Autodesk Fusion 360 part; units mm, degrees
(part 5 of 7)
sketch "Full-depth inlet-to-outlet bypass barrier sketch" plane through (0, 0, 4.9) normal (0, 0, 1) x (1, 0, 0) in component "Chamber / A3 top manifold with serial return"
  line L0 (4.9, 158) -> (27.25, 158)
  line L1 (27.25, 158) -> (27.25, 162.6)
  line L2 (27.25, 162.6) -> (4.9, 162.6)
  line L3 (4.9, 162.6) -> (4.9, 158)
  dimension "d1577" = 4.9
  dimension "d1578" = 158
  dimension "d1579" = 22.35
  dimension "d1580" = 4.6
  constraint horizontal L0
  constraint vertical L1
  constraint horizontal L2
  constraint vertical L3
  measures "d1577" horizontal distance of origin L0.start
  measures "d1578" vertical distance of origin L0.start
  measures "d1579" horizontal distance of L0.start L0.end
  measures "d1580" vertical distance of L0.end L1.end
extrude "Full-depth inlet-to-outlet bypass barrier" add sketch "Full-depth inlet-to-outlet bypass barrier sketch" along normal blind 31.1 contours L0 L1 L2 L3 picked at (12.35, 161.066667) bodies 74 in component "Chamber / A3 top manifold with serial return"
ref_plane "WorkPlane9" through (0, 0, 4.9) normal (0, 0, 1) x (1, 0, 0) in component "Chamber / A3 top manifold with serial return"
sketch "Exhaust junction upper 2 mm wall extension sketch" plane through (0, 0, 4.9) normal (0, 0, 1) x (1, 0, 0) in component "Chamber / A3 top manifold with serial return"
  line L0 (4.9, 162.5) -> (12.1, 162.5)
  line L1 (12.1, 162.5) -> (12.1, 167)
  line L2 (12.1, 167) -> (4.9, 167)
  line L3 (4.9, 167) -> (4.9, 162.5)
  dimension "d1585" = 4.9
  dimension "d1586" = 162.5
  dimension "d1587" = 7.2
  dimension "d1588" = 4.5
  constraint horizontal L0
  constraint vertical L1
  constraint horizontal L2
  constraint vertical L3
  measures "d1585" horizontal distance of origin L0.start
  measures "d1586" vertical distance of origin L0.start
  measures "d1587" horizontal distance of L0.start L0.end
  measures "d1588" vertical distance of L0.end L1.end
extrude "Exhaust junction upper 2 mm wall extension" add sketch "Exhaust junction upper 2 mm wall extension sketch" along normal blind 31.1 contours L0 L1 L2 L3 picked at (9.7, 164) bodies 74 in component "Chamber / A3 top manifold with serial return"
ref_plane "WorkPlane10" through (0, 0, 29) normal (0, 0, 1) x (1, 0, 0) in component "Chamber / A3 top manifold with serial return"
sketch "Rear return isolation above sensing-face sweep sketch" plane through (0, 0, 29) normal (0, 0, 1) x (1, 0, 0) in component "Chamber / A3 top manifold with serial return"
  line L0 (4.9, 149) -> (27.25, 149)
  line L1 (27.25, 149) -> (27.25, 158.1)
  line L2 (27.25, 158.1) -> (4.9, 158.1)
  line L3 (4.9, 158.1) -> (4.9, 149)
  dimension "d1593" = 4.9
  dimension "d1594" = 149
  dimension "d1595" = 22.35
  dimension "d1596" = 9.1
  constraint horizontal L0
  constraint vertical L1
  constraint horizontal L2
  constraint vertical L3
  measures "d1593" horizontal distance of origin L0.start
  measures "d1594" vertical distance of origin L0.start
  measures "d1595" horizontal distance of L0.start L0.end
  measures "d1596" vertical distance of L0.end L1.end
extrude "Rear return isolation above sensing-face sweep" add sketch "Rear return isolation above sensing-face sweep sketch" along normal blind 7 contours L0 L1 L2 L3 picked at (12.35, 152.033333) bodies 74 in component "Chamber / A3 top manifold with serial return"
ref_plane "WorkPlane11" through (0, 0, 28) normal (0, 0, 1) x (1, 0, 0) in component "Chamber / A3 top manifold with serial return"
sketch "Humidity compartment rear bypass baffle sketch" plane through (0, 0, 28) normal (0, 0, 1) x (1, 0, 0) in component "Chamber / A3 top manifold with serial return"
  line L0 (48, 162.4) -> (50, 162.4)
  line L1 (50, 162.4) -> (50, 175.1)
  line L2 (50, 175.1) -> (48, 175.1)
  line L3 (48, 175.1) -> (48, 162.4)
  dimension "d1601" = 48
  dimension "d1602" = 162.4
  dimension "d1603" = 2
  dimension "d1604" = 12.7
  constraint horizontal L0
  constraint vertical L1
  constraint horizontal L2
  constraint vertical L3
  measures "d1601" horizontal distance of origin L0.start
  measures "d1602" vertical distance of origin L0.start
  measures "d1603" horizontal distance of L0.start L0.end
  measures "d1604" vertical distance of L0.end L1.end
extrude "Humidity compartment rear bypass baffle" add sketch "Humidity compartment rear bypass baffle sketch" along normal blind 8 contours L0 L1 L2 L3 picked at (48.666667, 166.633333) bodies 74 in component "Chamber / A3 top manifold with serial return"
ref_plane "WorkPlane12" through (70.65, 0, 0) normal (1, 0, 0) x (0, 1, 0) in component "Chamber / A3 top manifold with serial return"
sketch "Inlet bore sketch" plane through (70.65, 0, 0) normal (1, 0, 0) x (0, 0, -1) in component "Chamber / A3 top manifold with serial return"
  circle A0 centre (-22, 162.5) radius 2.5
  dimension "d1610" = 162.5
  dimension "d1611" = 2.5
  measures "d1610" vertical distance of origin A0.centre
  measures "d1611" radius of A0
extrude "Inlet bore" cut sketch "Inlet bore sketch" along normal blind 11.45 contours A0 picked at (-21.937725, 164.26987) bodies 74 in component "Chamber / A3 top manifold with serial return"
ref_plane "WorkPlane13" through (0, 162.4, 0) normal (0, 1, 0) x (0, 0, 1) in component "Chamber / A3 top manifold with serial return"
sketch "Inlet rise bore sketch" plane through (0, 162.4, 0) normal (0, 1, 0) x (1, 0, 0) in component "Chamber / A3 top manifold with serial return"
  circle A0 centre (70.75, -22) radius 2.5
  dimension "d1616" = 70.75
  dimension "d1618" = 2.5
  measures "d1616" horizontal distance of origin A0.centre
  measures "d1618" radius of A0
extrude "Inlet rise bore" cut sketch "Inlet rise bore sketch" along normal blind 2.7 contours A0 picked at (70.581043, -23.369363) bodies 74 in component "Chamber / A3 top manifold with serial return"
ref_plane "WorkPlane14" through (67.9, 0, 0) normal (1, 0, 0) x (0, 1, 0) in component "Chamber / A3 top manifold with serial return"
sketch "Upper inlet turn bore sketch" plane through (67.9, 0, 0) normal (1, 0, 0) x (0, 0, -1) in component "Chamber / A3 top manifold with serial return"
  circle A0 centre (-22, 165) radius 2.5
  dimension "d1624" = 165
  dimension "d1625" = 2.5
  measures "d1624" vertical distance of origin A0.centre
  measures "d1625" radius of A0
extrude "Upper inlet turn bore" cut sketch "Upper inlet turn bore sketch" along normal blind 2.95 contours A0 picked at (-21.937725, 166.76987) bodies 74 in component "Chamber / A3 top manifold with serial return"
ref_plane "WorkPlane15" through (2.9, 0, 0) normal (1, 0, 0) x (0, 1, 0) in component "Chamber / A3 top manifold with serial return"
sketch "Exhaust wall and return junction bore sketch" plane through (2.9, 0, 0) normal (1, 0, 0) x (0, 0, -1) in component "Chamber / A3 top manifold with serial return"
  circle A0 centre (-22, 162.5) radius 2.5
  dimension "d1631" = 162.5
  dimension "d1632" = 2.5
  measures "d1631" vertical distance of origin A0.centre
  measures "d1632" radius of A0
extrude "Exhaust wall and return junction bore" cut sketch "Exhaust wall and return junction bore sketch" along normal blind 4.7 contours A0 picked at (-21.937725, 164.26987) bodies 74 in component "Chamber / A3 top manifold with serial return"
ref_plane "WorkPlane16" through (0, 0, 21.9) normal (0, 0, 1) x (1, 0, 0) in component "Chamber / A3 top manifold with serial return"
sketch "Exhaust return depth bore sketch" plane through (0, 0, 21.9) normal (0, 0, 1) x (1, 0, 0) in component "Chamber / A3 top manifold with serial return"
  circle A0 centre (7.5, 162.5) radius 2.5
  dimension "d1637" = 7.5
  dimension "d1638" = 162.5
  dimension "d1639" = 2.5
  measures "d1637" horizontal distance of origin A0.centre
  measures "d1638" vertical distance of origin A0.centre
  measures "d1639" radius of A0
extrude "Exhaust return depth bore" cut sketch "Exhaust return depth bore sketch" along normal blind 11.7 contours A0 picked at (7.562275, 160.73013) bodies 74 in component "Chamber / A3 top manifold with serial return"
ref_plane "WorkPlane17" through (0, 145.4, 0) normal (0, 1, 0) x (0, 0, 1) in component "Chamber / A3 top manifold with serial return"
sketch "Exhaust return from below face-sweep barrier sketch" plane through (0, 145.4, 0) normal (0, 1, 0) x (1, 0, 0) in component "Chamber / A3 top manifold with serial return"
  circle A0 centre (7.5, -33.5) radius 2.5
  dimension "d1644" = 7.5
  dimension "d1645" = 33.5
  dimension "d1646" = 2.5
  measures "d1644" horizontal distance of origin A0.centre
  measures "d1645" vertical distance of origin A0.centre
  measures "d1646" radius of A0
extrude "Exhaust return from below face-sweep barrier" cut sketch "Exhaust return from below face-sweep barrier sketch" along normal blind 17.2 contours A0 picked at (8.260115, -33.985772) bodies 74 in component "Chamber / A3 top manifold with serial return"
ref_plane "WorkPlane18" through (32.9, 0, 0) normal (1, 0, 0) x (0, 1, 0) in component "Chamber / A3 top manifold with serial return"
sketch "AO2 nose clearance through wet wall sketch" plane through (32.9, 0, 0) normal (1, 0, 0) x (0, 0, -1) in component "Chamber / A3 top manifold with serial return"
  circle A0 centre (-21.75, 142.5) radius 8.1
  dimension "d1651" = 21.75
  dimension "d1652" = 142.5
  dimension "d1653" = 8.1
  measures "d1651" horizontal distance of origin A0.centre
  measures "d1652" vertical distance of origin A0.centre
  measures "d1653" radius of A0
extrude "AO2 nose clearance through wet wall" cut sketch "AO2 nose clearance through wet wall sketch" along normal blind 2.2 contours A0 picked at (-19.663035, 144.610945) bodies 74 in component "Chamber / A3 top manifold with serial return"
ref_plane "WorkPlane19" through (0, 0, 30) normal (0, 0, 1) x (1, 0, 0) in component "Chamber / A3 top manifold with serial return"
sketch "M2 lid insert boss sketch" plane through (0, 0, 30) normal (0, 0, 1) x (1, 0, 0) in component "Chamber / A3 top manifold with serial return"
  circle A0 centre (18, 159) radius 3.6
  dimension "d1658" = 18
  dimension "d1659" = 159
  dimension "d1660" = 3.6
  measures "d1658" horizontal distance of origin A0.centre
  measures "d1659" vertical distance of origin A0.centre
  measures "d1660" radius of A0
extrude "M2 lid insert boss" add sketch "M2 lid insert boss sketch" along normal blind 6 contours A0 picked at (17.732975, 161.211234) bodies 74 in component "Chamber / A3 top manifold with serial return"
ref_plane "WorkPlane20" through (0, 0, 32) normal (0, 0, 1) x (1, 0, 0) in component "Chamber / A3 top manifold with serial return"
sketch "M2 blind pilot with 2 mm nominal floor sketch" plane through (0, 0, 32) normal (0, 0, 1) x (1, 0, 0) in component "Chamber / A3 top manifold with serial return"
  circle A0 centre (18, 159) radius 1.6
  dimension "d1665" = 18
  dimension "d1666" = 159
  dimension "d1667" = 1.6
  measures "d1665" horizontal distance of origin A0.centre
  measures "d1666" vertical distance of origin A0.centre
  measures "d1667" radius of A0
extrude "M2 blind pilot with 2 mm nominal floor" cut sketch "M2 blind pilot with 2 mm nominal floor sketch" along normal blind 4.1 contours A0 picked at (17.371683, 159.362759) bodies 74 in component "Chamber / A3 top manifold with serial return"
ref_plane "WorkPlane21" through (0, 0, 30) normal (0, 0, 1) x (1, 0, 0) in component "Chamber / A3 top manifold with serial return"
sketch "M2 lid insert boss sketch (1)" plane through (0, 0, 30) normal (0, 0, 1) x (1, 0, 0) in component "Chamber / A3 top manifold with serial return"
  circle A0 centre (30.5, 135) radius 3.6
  dimension "d1672" = 30.5
  dimension "d1673" = 135
  dimension "d1674" = 3.6
  measures "d1672" horizontal distance of origin A0.centre
  measures "d1673" vertical distance of origin A0.centre
  measures "d1674" radius of A0
extrude "M2 lid insert boss (1)" add sketch "M2 lid insert boss sketch (1)" along normal blind 6 contours A0 picked at (30.232975, 137.211234) bodies 74 in component "Chamber / A3 top manifold with serial return"
ref_plane "WorkPlane22" through (0, 0, 32) normal (0, 0, 1) x (1, 0, 0) in component "Chamber / A3 top manifold with serial return"
sketch "M2 blind pilot with 2 mm nominal floor sketch (1)" plane through (0, 0, 32) normal (0, 0, 1) x (1, 0, 0) in component "Chamber / A3 top manifold with serial return"
  circle A0 centre (30.5, 135) radius 1.6
  dimension "d1679" = 30.5
  dimension "d1680" = 135
  dimension "d1681" = 1.6
  measures "d1679" horizontal distance of origin A0.centre
  measures "d1680" vertical distance of origin A0.centre
  measures "d1681" radius of A0
extrude "M2 blind pilot with 2 mm nominal floor (1)" cut sketch "M2 blind pilot with 2 mm nominal floor sketch (1)" along normal blind 4.1 contours A0 picked at (30.233333, 135.46188) bodies 74 in component "Chamber / A3 top manifold with serial return"
ref_plane "WorkPlane23" through (0, 0, 30) normal (0, 0, 1) x (1, 0, 0) in component "Chamber / A3 top manifold with serial return"
sketch "M2 lid insert boss sketch (2)" plane through (0, 0, 30) normal (0, 0, 1) x (1, 0, 0) in component "Chamber / A3 top manifold with serial return"
  circle A0 centre (17, 172.2) radius 3.6
  dimension "d1686" = 17
  dimension "d1687" = 172.2
  dimension "d1688" = 3.6
  measures "d1686" horizontal distance of origin A0.centre
  measures "d1687" vertical distance of origin A0.centre
  measures "d1688" radius of A0
extrude "M2 lid insert boss (2)" add sketch "M2 lid insert boss sketch (2)" along normal blind 6 contours A0 picked at (16.732975, 169.988766) bodies 74 in component "Chamber / A3 top manifold with serial return"
ref_plane "WorkPlane24" through (0, 0, 32) normal (0, 0, 1) x (1, 0, 0) in component "Chamber / A3 top manifold with serial return"
sketch "M2 blind pilot with 2 mm nominal floor sketch (2)" plane through (0, 0, 32) normal (0, 0, 1) x (1, 0, 0) in component "Chamber / A3 top manifold with serial return"
  circle A0 centre (17, 172.2) radius 1.6
  dimension "d1693" = 17
  dimension "d1694" = 172.2
  dimension "d1695" = 1.6
  measures "d1693" horizontal distance of origin A0.centre
  measures "d1694" vertical distance of origin A0.centre
  measures "d1695" radius of A0
extrude "M2 blind pilot with 2 mm nominal floor (2)" cut sketch "M2 blind pilot with 2 mm nominal floor sketch (2)" along normal blind 4.1 contours A0 picked at (16.733333, 172.66188) bodies 74 in component "Chamber / A3 top manifold with serial return"
ref_plane "WorkPlane25" through (0, 0, 30) normal (0, 0, 1) x (1, 0, 0) in component "Chamber / A3 top manifold with serial return"
sketch "M2 lid insert boss sketch (3)" plane through (0, 0, 30) normal (0, 0, 1) x (1, 0, 0) in component "Chamber / A3 top manifold with serial return"
  circle A0 centre (68, 172.2) radius 3.6
  dimension "d1700" = 68
  dimension "d1701" = 172.2
  dimension "d1702" = 3.6
  measures "d1700" horizontal distance of origin A0.centre
  measures "d1701" vertical distance of origin A0.centre
  measures "d1702" radius of A0
extrude "M2 lid insert boss (3)" add sketch "M2 lid insert boss sketch (3)" along normal blind 6 contours A0 picked at (69.110324, 171.003355) bodies 74 in component "Chamber / A3 top manifold with serial return"
ref_plane "WorkPlane26" through (0, 0, 32) normal (0, 0, 1) x (1, 0, 0) in component "Chamber / A3 top manifold with serial return"
sketch "M2 blind pilot with 2 mm nominal floor sketch (3)" plane through (0, 0, 32) normal (0, 0, 1) x (1, 0, 0) in component "Chamber / A3 top manifold with serial return"
  circle A0 centre (68, 172.2) radius 1.6
  dimension "d1707" = 68
  dimension "d1708" = 172.2
  dimension "d1709" = 1.6
  measures "d1707" horizontal distance of origin A0.centre
  measures "d1708" vertical distance of origin A0.centre
  measures "d1709" radius of A0
extrude "M2 blind pilot with 2 mm nominal floor (3)" cut sketch "M2 blind pilot with 2 mm nominal floor sketch (3)" along normal blind 4.1 contours A0 picked at (68.480517, 171.968595) bodies 74 in component "Chamber / A3 top manifold with serial return"
ref_plane "WorkPlane27" through (0, 130, 0) normal (0, 1, 0) x (0, 0, 1) in component "Chamber / A3 top manifold with serial return"
sketch "Feedthrough support collar sketch" plane through (0, 130, 0) normal (0, 1, 0) x (1, 0, 0) in component "Chamber / A3 top manifold with serial return"
  circle A0 centre (17, -31.5) radius 4.2
  dimension "d1714" = 17
  dimension "d1715" = 31.5
  dimension "d1716" = 4.2
  measures "d1714" horizontal distance of origin A0.centre
  measures "d1715" vertical distance of origin A0.centre
  measures "d1716" radius of A0
extrude "Feedthrough support collar" add sketch "Feedthrough support collar sketch" along normal blind 2 contours A0 picked at (16.583849, -32.170777) bodies 74 in component "Chamber / A3 top manifold with serial return"
ref_plane "WorkPlane28" through (0, 129.9, 0) normal (0, 1, 0) x (0, 0, 1) in component "Chamber / A3 top manifold with serial return"
sketch "Feedthrough seal seat sketch" plane through (0, 129.9, 0) normal (0, 1, 0) x (1, 0, 0) in component "Chamber / A3 top manifold with serial return"
  circle A0 centre (17, -31.5) radius 2.2
  dimension "d1721" = 17
  dimension "d1722" = 31.5
  dimension "d1723" = 2.2
  measures "d1721" horizontal distance of origin A0.centre
  measures "d1722" vertical distance of origin A0.centre
  measures "d1723" radius of A0
extrude "Feedthrough seal seat" cut sketch "Feedthrough seal seat sketch" along normal blind 2.2 contours A0 picked at (17.227614, -32.642426) bodies 74 in component "Chamber / A3 top manifold with serial return"
ref_plane "WorkPlane1" through (0, 0, 36) normal (0, 0, 1) x (1, 0, 0) in component "Chamber / A3 four-screw service lid"
sketch "Lid CO pocket sketch" plane through (0, 0, 36) normal (0, 0, 1) x (1, 0, 0) in component "Chamber / A3 four-screw service lid"
  line L0 (3, 130) -> (35, 130)
  line L1 (35, 130) -> (35, 167)
  line L2 (35, 167) -> (3, 167)
  line L3 (3, 167) -> (3, 130)
  dimension "d1728" = 3
  dimension "d1729" = 130
  dimension "d1730" = 32
  dimension "d1731" = 37
  constraint horizontal L0
  constraint vertical L1
  constraint horizontal L2
  constraint vertical L3
  measures "d1728" horizontal distance of origin L0.start
  measures "d1729" vertical distance of origin L0.start
  measures "d1730" horizontal distance of L0.start L0.end
  measures "d1731" vertical distance of L0.end L1.end
extrude "Lid CO pocket" add sketch "Lid CO pocket sketch" along normal blind 2 separate body contours L0 L1 L2 L3 picked at (13.666667, 142.333333) makes body 75 in component "Chamber / A3 four-screw service lid"
ref_plane "WorkPlane2" through (0, 0, 36) normal (0, 0, 1) x (1, 0, 0) in component "Chamber / A3 four-screw service lid"
sketch "Lid upper row sketch" plane through (0, 0, 36) normal (0, 0, 1) x (1, 0, 0) in component "Chamber / A3 four-screw service lid"
  line L0 (13, 160.5) -> (72.5, 160.5)
  line L1 (72.5, 160.5) -> (72.5, 177)
  line L2 (72.5, 177) -> (13, 177)
  line L3 (13, 177) -> (13, 160.5)
  dimension "d1736" = 13
  dimension "d1737" = 160.5
  dimension "d1738" = 59.5
  dimension "d1739" = 16.5
  constraint horizontal L0
  constraint vertical L1
  constraint horizontal L2
  constraint vertical L3
  measures "d1736" horizontal distance of origin L0.start
  measures "d1737" vertical distance of origin L0.start
  measures "d1738" horizontal distance of L0.start L0.end
  measures "d1739" vertical distance of L0.end L1.end
extrude "Lid upper row" add sketch "Lid upper row sketch" along normal blind 2 contours L0 L1 L2 L3 picked at (32.833333, 171.5) bodies 75 in component "Chamber / A3 four-screw service lid"
ref_plane "WorkPlane3" through (0, 0, 35.9) normal (0, 0, 1) x (1, 0, 0) in component "Chamber / A3 four-screw service lid"
sketch "M2 lid clearance sketch" plane through (0, 0, 35.9) normal (0, 0, 1) x (1, 0, 0) in component "Chamber / A3 four-screw service lid"
  circle A0 centre (18, 159) radius 1.1
  dimension "d1744" = 18
  dimension "d1745" = 159
  dimension "d1746" = 1.1
  measures "d1744" horizontal distance of origin A0.centre
  measures "d1745" vertical distance of origin A0.centre
  measures "d1746" radius of A0
extrude "M2 lid clearance" cut sketch "M2 lid clearance sketch" along normal blind 2.2 contours A0 picked at (18.133958, 158.767977) bodies 75 in component "Chamber / A3 four-screw service lid"
ref_plane "WorkPlane4" through (0, 0, 35.9) normal (0, 0, 1) x (1, 0, 0) in component "Chamber / A3 four-screw service lid"
sketch "M2 lid clearance sketch (1)" plane through (0, 0, 35.9) normal (0, 0, 1) x (1, 0, 0) in component "Chamber / A3 four-screw service lid"
  circle A0 centre (30.5, 135) radius 1.1
  dimension "d1751" = 30.5
  dimension "d1752" = 135
  dimension "d1753" = 1.1
  measures "d1751" horizontal distance of origin A0.centre
  measures "d1752" vertical distance of origin A0.centre
  measures "d1753" radius of A0
extrude "M2 lid clearance (1)" cut sketch "M2 lid clearance sketch (1)" along normal blind 2.2 contours A0 picked at (30.460696, 135.286672) bodies 75 in component "Chamber / A3 four-screw service lid"
ref_plane "WorkPlane5" through (0, 0, 35.9) normal (0, 0, 1) x (1, 0, 0) in component "Chamber / A3 four-screw service lid"
sketch "M2 lid clearance sketch (2)" plane through (0, 0, 35.9) normal (0, 0, 1) x (1, 0, 0) in component "Chamber / A3 four-screw service lid"
  circle A0 centre (17, 172.2) radius 1.1
  dimension "d1758" = 17
  dimension "d1759" = 172.2
  dimension "d1760" = 1.1
  measures "d1758" horizontal distance of origin A0.centre
  measures "d1759" vertical distance of origin A0.centre
  measures "d1760" radius of A0
extrude "M2 lid clearance (2)" cut sketch "M2 lid clearance sketch (2)" along normal blind 2.2 contours A0 picked at (17.133958, 171.967977) bodies 75 in component "Chamber / A3 four-screw service lid"
ref_plane "WorkPlane6" through (0, 0, 35.9) normal (0, 0, 1) x (1, 0, 0) in component "Chamber / A3 four-screw service lid"
sketch "M2 lid clearance sketch (3)" plane through (0, 0, 35.9) normal (0, 0, 1) x (1, 0, 0) in component "Chamber / A3 four-screw service lid"
  circle A0 centre (68, 172.2) radius 1.1
  dimension "d1765" = 68
  dimension "d1766" = 172.2
  dimension "d1767" = 1.1
  measures "d1765" horizontal distance of origin A0.centre
  measures "d1766" vertical distance of origin A0.centre
  measures "d1767" radius of A0
extrude "M2 lid clearance (3)" cut sketch "M2 lid clearance sketch (3)" along normal blind 2.2 contours A0 picked at (68.183333, 171.882457) bodies 75 in component "Chamber / A3 four-screw service lid"
ref_plane "WorkPlane1" through (35, 0, 0) normal (1, 0, 0) x (0, 1, 0) in component "Chamber / AO2 hand-tight adapter reference"
sketch "Hand-tight adapter shoulder sketch" plane through (35, 0, 0) normal (1, 0, 0) x (0, 0, -1) in component "Chamber / AO2 hand-tight adapter reference"
  circle A0 centre (-21.75, 142.5) radius 10.1
  dimension "d1772" = 21.75
  dimension "d1773" = 142.5
  dimension "d1774" = 10.1
  measures "d1772" horizontal distance of origin A0.centre
  measures "d1773" vertical distance of origin A0.centre
  measures "d1774" radius of A0
extrude "Hand-tight adapter shoulder" add sketch "Hand-tight adapter shoulder sketch" along normal blind 3.8 separate body contours A0 picked at (-24.531671, 144.396511) makes body 76 in component "Chamber / AO2 hand-tight adapter reference"
ref_plane "WorkPlane2" through (34.9, 0, 0) normal (1, 0, 0) x (0, 1, 0) in component "Chamber / AO2 hand-tight adapter reference"
sketch "Simplified female M16 clearance surface sketch" plane through (34.9, 0, 0) normal (1, 0, 0) x (0, 0, -1) in component "Chamber / AO2 hand-tight adapter reference"
  circle A0 centre (-21.75, 142.5) radius 8.1
  dimension "d1779" = 21.75
  dimension "d1780" = 142.5
  dimension "d1781" = 8.1
  measures "d1779" horizontal distance of origin A0.centre
  measures "d1780" vertical distance of origin A0.centre
  measures "d1781" radius of A0
extrude "Simplified female M16 clearance surface" cut sketch "Simplified female M16 clearance surface sketch" along normal blind 4 contours A0 picked at (-19.663035, 144.610945) bodies 76 in component "Chamber / AO2 hand-tight adapter reference"
ref_plane "WorkPlane1" through (39, 0, 0) normal (1, 0, 0) x (0, 1, 0) in component "Sensor / AO2 dry body with wetted threaded nose"
sketch "Sketch1" plane through (39, 0, 0) normal (1, 0, 0) x (0, 0, -1) in component "Sensor / AO2 dry body with wetted threaded nose"
  circle A0 centre (-21.75, 142.5) radius 14.65
  dimension "d1786" = 21.75
  dimension "d1787" = 142.5
  dimension "d1788" = 14.65
  measures "d1786" horizontal distance of origin A0.centre
  measures "d1787" vertical distance of origin A0.centre
  measures "d1788" radius of A0
extrude "AO2 Ø29.3 dry body" add sketch "Sketch1" along normal blind 31.75 separate body contours A0 picked at (-17.618648, 133.921158) makes body 77 in component "Sensor / AO2 dry body with wetted threaded nose"
ref_plane "WorkPlane2" through (32.5, 0, 0) normal (1, 0, 0) x (0, 1, 0) in component "Sensor / AO2 dry body with wetted threaded nose"
sketch "AO2 nominal threaded nose sketch" plane through (32.5, 0, 0) normal (1, 0, 0) x (0, 0, -1) in component "Sensor / AO2 dry body with wetted threaded nose"
  circle A0 centre (-21.75, 142.5) radius 8
  dimension "d1793" = 21.75
  dimension "d1794" = 142.5
  dimension "d1795" = 8
  measures "d1793" horizontal distance of origin A0.centre
  measures "d1794" vertical distance of origin A0.centre
  measures "d1795" radius of A0
extrude "AO2 nominal threaded nose" add sketch "AO2 nominal threaded nose sketch" along normal blind 6.5 contours A0 picked at (-25.326107, 141.166097) bodies 77 in component "Sensor / AO2 dry body with wetted threaded nose"
ref_plane "WorkPlane1" through (0, 0, 16.75) normal (0, 0, 1) x (1, 0, 0) in component "Sensor / AO2 cable connector allowance"
sketch "AO2 connector and wire origin allowance sketch" plane through (0, 0, 16.75) normal (0, 0, 1) x (1, 0, 0) in component "Sensor / AO2 cable connector allowance"
  line L0 (70.75, 137.5) -> (77.25, 137.5)
  line L1 (77.25, 137.5) -> (77.25, 147.5)
  line L2 (77.25, 147.5) -> (70.75, 147.5)
  line L3 (70.75, 147.5) -> (70.75, 137.5)
  dimension "d1800" = 70.75
  dimension "d1801" = 137.5
  dimension "d1802" = 6.5
  dimension "d1803" = 10
  constraint horizontal L0
  constraint vertical L1
  constraint horizontal L2
  constraint vertical L3
  measures "d1800" horizontal distance of origin L0.start
  measures "d1801" vertical distance of origin L0.start
  measures "d1802" horizontal distance of L0.start L0.end
  measures "d1803" vertical distance of L0.end L1.end
extrude "AO2 connector and wire origin allowance" add sketch "AO2 connector and wire origin allowance sketch" along normal blind 10 separate body contours L0 L1 L2 L3 picked at (72.916667, 144.166667) makes body 78 in component "Sensor / AO2 cable connector allowance"
ref_plane "WorkPlane1" through (0, 0, 5.4) normal (0, 0, 1) x (1, 0, 0) in component "Sensor / ZE07-CO drawing-derived assembly"
sketch "ZE07 PCB sketch" plane through (0, 0, 5.4) normal (0, 0, 1) x (1, 0, 0) in component "Sensor / ZE07-CO drawing-derived assembly"
  line L0 (8.95, 132.3) -> (10.55, 132.3)
  line L1 (10.55, 132.3) -> (10.55, 157.7)
  line L2 (10.55, 157.7) -> (8.95, 157.7)
  line L3 (8.95, 157.7) -> (8.95, 132.3)
  dimension "d1808" = 8.95
  dimension "d1809" = 132.3
  dimension "d1810" = 1.6
  dimension "d1811" = 25.4
  constraint horizontal L0
  constraint vertical L1
  constraint horizontal L2
  constraint vertical L3
  measures "d1808" horizontal distance of origin L0.start
  measures "d1809" vertical distance of origin L0.start
  measures "d1810" horizontal distance of L0.start L0.end
  measures "d1811" vertical distance of L0.end L1.end
extrude "ZE07 PCB" add sketch "ZE07 PCB sketch" along normal blind 22.4 separate body contours L0 L1 L2 L3 picked at (9.483333, 149.233333) makes body 79 in component "Sensor / ZE07-CO drawing-derived assembly"
ref_plane "WorkPlane2" through (10.55, 0, 0) normal (1, 0, 0) x (0, 1, 0) in component "Sensor / ZE07-CO drawing-derived assembly"
sketch "ZE07 CO can sketch" plane through (10.55, 0, 0) normal (1, 0, 0) x (0, 0, -1) in component "Sensor / ZE07-CO drawing-derived assembly"
  circle A0 centre (-16.6, 145) radius 10
  dimension "d1816" = 16.6
  dimension "d1817" = 145
  dimension "d1818" = 10
  measures "d1816" horizontal distance of origin A0.centre
  measures "d1817" vertical distance of origin A0.centre
  measures "d1818" radius of A0
extrude "ZE07 CO can" add sketch "ZE07 CO can sketch" along normal blind 16.7 separate body contours A0 picked at (-13.59677, 143.553721) makes body 80 in component "Sensor / ZE07-CO drawing-derived assembly"
ref_plane "WorkPlane3" through (0, 0, 13.4) normal (0, 0, 1) x (1, 0, 0) in component "Sensor / ZE07-CO drawing-derived assembly"
sketch "ZE07 header envelope sketch" plane through (0, 0, 13.4) normal (0, 0, 1) x (1, 0, 0) in component "Sensor / ZE07-CO drawing-derived assembly"
  line L0 (5.5, 134.3) -> (8.95, 134.3)
  line L1 (8.95, 134.3) -> (8.95, 140.3)
  line L2 (8.95, 140.3) -> (5.5, 140.3)
  line L3 (5.5, 140.3) -> (5.5, 134.3)
  dimension "d1823" = 5.5
  dimension "d1824" = 134.3
  dimension "d1825" = 3.45
  dimension "d1826" = 6
  constraint horizontal L0
  constraint vertical L1
  constraint horizontal L2
  constraint vertical L3
  measures "d1823" horizontal distance of origin L0.start
  measures "d1824" vertical distance of origin L0.start
  measures "d1825" horizontal distance of L0.start L0.end
  measures "d1826" vertical distance of L0.end L1.end
extrude "ZE07 header envelope" add sketch "ZE07 header envelope sketch" along normal blind 8 separate body contours L0 L1 L2 L3 picked at (7.8, 138.3) makes body 81 in component "Sensor / ZE07-CO drawing-derived assembly"
ref_plane "WorkPlane1" through (0, 0, 8) normal (0, 0, 1) x (1, 0, 0) in component "Sensor / MD62 body and full-length lead references"
sketch "MD62 full-size body sketch" plane through (0, 0, 8) normal (0, 0, 1) x (1, 0, 0) in component "Sensor / MD62 body and full-length lead references"
  line L0 (19, 163) -> (33, 163)
  line L1 (33, 163) -> (33, 172.5)
  line L2 (33, 172.5) -> (19, 172.5)
  line L3 (19, 172.5) -> (19, 163)
  dimension "d1831" = 19
  dimension "d1832" = 163
  dimension "d1833" = 14
  dimension "d1834" = 9.5
  constraint horizontal L0
  constraint vertical L1
  constraint horizontal L2
  constraint vertical L3
  measures "d1831" horizontal distance of origin L0.start
  measures "d1832" vertical distance of origin L0.start
  measures "d1833" horizontal distance of L0.start L0.end
  measures "d1834" vertical distance of L0.end L1.end
extrude "MD62 full-size body" add sketch "MD62 full-size body sketch" along normal blind 19 separate body contours L0 L1 L2 L3 picked at (23.666667, 169.333333) makes body 82 in component "Sensor / MD62 body and full-length lead references"
ref_plane "WorkPlane2" through (33, 0, 0) normal (1, 0, 0) x (0, 1, 0) in component "Sensor / MD62 body and full-length lead references"
sketch "MD62 full-length lead visual reference sketch" plane through (33, 0, 0) normal (1, 0, 0) x (0, 0, -1) in component "Sensor / MD62 body and full-length lead references"
  circle A0 centre (-13, 164.2) radius 0.25
  dimension "d1839" = 13
  dimension "d1840" = 164.2
  dimension "d1841" = 0.25
  measures "d1839" horizontal distance of origin A0.centre
  measures "d1840" vertical distance of origin A0.centre
  measures "d1841" radius of A0
extrude "MD62 full-length lead visual reference" add sketch "MD62 full-length lead visual reference sketch" along normal blind 27 separate body contours A0 picked at (-12.981457, 164.118756) makes body 83 in component "Sensor / MD62 body and full-length lead references"
ref_plane "WorkPlane3" through (33, 0, 0) normal (1, 0, 0) x (0, 1, 0) in component "Sensor / MD62 body and full-length lead references"
sketch "MD62 full-length lead visual reference sketch (1)" plane through (33, 0, 0) normal (1, 0, 0) x (0, 0, -1) in component "Sensor / MD62 body and full-length lead references"
  circle A0 centre (-24, 164.2) radius 0.25
  dimension "d1846" = 24
  dimension "d1847" = 164.2
  dimension "d1848" = 0.25
  measures "d1846" horizontal distance of origin A0.centre
  measures "d1847" vertical distance of origin A0.centre
  measures "d1848" radius of A0
extrude "MD62 full-length lead visual reference (1)" add sketch "MD62 full-length lead visual reference sketch (1)" along normal blind 27 separate body contours A0 picked at (-23.981457, 164.118756) makes body 84 in component "Sensor / MD62 body and full-length lead references"
ref_plane "WorkPlane4" through (33, 0, 0) normal (1, 0, 0) x (0, 1, 0) in component "Sensor / MD62 body and full-length lead references"
sketch "MD62 full-length lead visual reference sketch (2)" plane through (33, 0, 0) normal (1, 0, 0) x (0, 0, -1) in component "Sensor / MD62 body and full-length lead references"
  circle A0 centre (-13, 171.3) radius 0.25
  dimension "d1853" = 13
  dimension "d1854" = 171.3
  dimension "d1855" = 0.25
  measures "d1853" horizontal distance of origin A0.centre
  measures "d1854" vertical distance of origin A0.centre
  measures "d1855" radius of A0
extrude "MD62 full-length lead visual reference (2)" add sketch "MD62 full-length lead visual reference sketch (2)" along normal blind 27 separate body contours A0 picked at (-12.981457, 171.218756) makes body 85 in component "Sensor / MD62 body and full-length lead references"
ref_plane "WorkPlane5" through (33, 0, 0) normal (1, 0, 0) x (0, 1, 0) in component "Sensor / MD62 body and full-length lead references"
sketch "MD62 full-length lead visual reference sketch (3)" plane through (33, 0, 0) normal (1, 0, 0) x (0, 0, -1) in component "Sensor / MD62 body and full-length lead references"
  circle A0 centre (-24, 171.3) radius 0.25
  dimension "d1860" = 24
  dimension "d1861" = 171.3
  dimension "d1862" = 0.25
  measures "d1860" horizontal distance of origin A0.centre
  measures "d1861" vertical distance of origin A0.centre
  measures "d1862" radius of A0
extrude "MD62 full-length lead visual reference (3)" add sketch "MD62 full-length lead visual reference sketch (3)" along normal blind 27 separate body contours A0 picked at (-23.981457, 171.218756) makes body 86 in component "Sensor / MD62 body and full-length lead references"
ref_plane "WorkPlane1" through (0, 0, 6) normal (0, 0, 1) x (1, 0, 0) in component "Sensor / GYBMEP humidity breakout reference"
sketch "GYBMEP provisional PCB sketch" plane through (0, 0, 6) normal (0, 0, 1) x (1, 0, 0) in component "Sensor / GYBMEP humidity breakout reference"
  line L0 (53, 162.8) -> (70, 162.8)
  line L1 (70, 162.8) -> (70, 174.8)
  line L2 (70, 174.8) -> (53, 174.8)
  line L3 (53, 174.8) -> (53, 162.8)
  dimension "d1867" = 53
  dimension "d1868" = 162.8
  dimension "d1869" = 17
  dimension "d1870" = 12
  constraint horizontal L0
  constraint vertical L1
  constraint horizontal L2
  constraint vertical L3
  measures "d1867" horizontal distance of origin L0.start
  measures "d1868" vertical distance of origin L0.start
  measures "d1869" horizontal distance of L0.start L0.end
  measures "d1870" vertical distance of L0.end L1.end
extrude "GYBMEP provisional PCB" add sketch "GYBMEP provisional PCB sketch" along normal blind 1.6 separate body contours L0 L1 L2 L3 picked at (58.666667, 170.8) makes body 87 in component "Sensor / GYBMEP humidity breakout reference"
ref_plane "WorkPlane2" through (0, 0, 7.6) normal (0, 0, 1) x (1, 0, 0) in component "Sensor / GYBMEP humidity breakout reference"
sketch "Humidity cap visual reference sketch" plane through (0, 0, 7.6) normal (0, 0, 1) x (1, 0, 0) in component "Sensor / GYBMEP humidity breakout reference"
  line L0 (65, 170) -> (68, 170)
  line L1 (68, 170) -> (68, 173)
  line L2 (68, 173) -> (65, 173)
  line L3 (65, 173) -> (65, 170)
  dimension "d1875" = 65
  dimension "d1876" = 170
  dimension "d1877" = 3
  dimension "d1878" = 3
  constraint horizontal L0
  constraint vertical L1
  constraint horizontal L2
  constraint vertical L3
  measures "d1875" horizontal distance of origin L0.start
  measures "d1876" vertical distance of origin L0.start
  measures "d1877" horizontal distance of L0.start L0.end
  measures "d1878" vertical distance of L0.end L1.end
extrude "Humidity cap visual reference" add sketch "Humidity cap visual reference sketch" along normal blind 1.2 separate body contours L0 L1 L2 L3 picked at (66, 172) makes body 88 in component "Sensor / GYBMEP humidity breakout reference"
ref_plane "WorkPlane3" through (0, 0, 7.6) normal (0, 0, 1) x (1, 0, 0) in component "Sensor / GYBMEP humidity breakout reference"
sketch "Breakout regulator height allowance sketch" plane through (0, 0, 7.6) normal (0, 0, 1) x (1, 0, 0) in component "Sensor / GYBMEP humidity breakout reference"
  line L0 (55, 165) -> (59, 165)
  line L1 (59, 165) -> (59, 170)
  line L2 (59, 170) -> (55, 170)
  line L3 (55, 170) -> (55, 165)
  dimension "d1883" = 55
  dimension "d1884" = 165
  dimension "d1885" = 4
  dimension "d1886" = 5
  constraint horizontal L0
  constraint vertical L1
  constraint horizontal L2
  constraint vertical L3
  measures "d1883" horizontal distance of origin L0.start
  measures "d1884" vertical distance of origin L0.start
  measures "d1885" horizontal distance of L0.start L0.end
  measures "d1886" vertical distance of L0.end L1.end
extrude "Breakout regulator height allowance" add sketch "Breakout regulator height allowance sketch" along normal blind 3.4 separate body contours L0 L1 L2 L3 picked at (56.333333, 168.333333) makes body 89 in component "Sensor / GYBMEP humidity breakout reference"
ref_plane "WorkPlane1" through (82, 0, 0) normal (1, 0, 0) x (0, 1, 0) in component "Gas / Viewer-left inlet fitting reference"
sketch "Viewer-left inlet OD8 tube reference sketch" plane through (82, 0, 0) normal (1, 0, 0) x (0, 0, -1) in component "Gas / Viewer-left inlet fitting reference"
  circle A0 centre (-22, 162.5) radius 4
  dimension "d1892" = 162.5
  dimension "d1893" = 4
  measures "d1892" vertical distance of origin A0.centre
  measures "d1893" radius of A0
extrude "Viewer-left inlet OD8 tube reference" add sketch "Viewer-left inlet OD8 tube reference sketch" along normal blind 9 separate body contours A0 picked at (-20.949792, 164.378416) makes body 90 in component "Gas / Viewer-left inlet fitting reference"
ref_plane "WorkPlane2" through (81.9, 0, 0) normal (1, 0, 0) x (0, 1, 0) in component "Gas / Viewer-left inlet fitting reference"
sketch "Viewer-left inlet ID5 bore sketch" plane through (81.9, 0, 0) normal (1, 0, 0) x (0, 0, -1) in component "Gas / Viewer-left inlet fitting reference"
  circle A0 centre (-22, 162.5) radius 2.5
  dimension "d1899" = 162.5
  dimension "d1900" = 2.5
  measures "d1899" vertical distance of origin A0.centre
  measures "d1900" radius of A0
extrude "Viewer-left inlet ID5 bore" cut sketch "Viewer-left inlet ID5 bore sketch" along normal blind 9.2 contours A0 picked at (-21.937725, 164.26987) bodies 90 in component "Gas / Viewer-left inlet fitting reference"
ref_plane "WorkPlane1" through (-6, 0, 0) normal (1, 0, 0) x (0, 1, 0) in component "Gas / Viewer-right exhaust fitting reference"
sketch "Viewer-right exhaust OD8 tube reference sketch" plane through (-6, 0, 0) normal (1, 0, 0) x (0, 0, -1) in component "Gas / Viewer-right exhaust fitting reference"
  circle A0 centre (-22, 162.5) radius 4
  dimension "d1906" = 162.5
  dimension "d1907" = 4
  measures "d1906" vertical distance of origin A0.centre
  measures "d1907" radius of A0
extrude "Viewer-right exhaust OD8 tube reference" add sketch "Viewer-right exhaust OD8 tube reference sketch" along normal blind 9 separate body contours A0 picked at (-20.949792, 164.378416) makes body 91 in component "Gas / Viewer-right exhaust fitting reference"
ref_plane "WorkPlane2" through (-6.1, 0, 0) normal (1, 0, 0) x (0, 1, 0) in component "Gas / Viewer-right exhaust fitting reference"
sketch "Viewer-right exhaust ID5 bore sketch" plane through (-6.1, 0, 0) normal (1, 0, 0) x (0, 0, -1) in component "Gas / Viewer-right exhaust fitting reference"
  circle A0 centre (-22, 162.5) radius 2.5
  dimension "d1913" = 162.5
  dimension "d1914" = 2.5
  measures "d1913" vertical distance of origin A0.centre
  measures "d1914" radius of A0
extrude "Viewer-right exhaust ID5 bore" cut sketch "Viewer-right exhaust ID5 bore sketch" along normal blind 9.2 contours A0 picked at (-21.937725, 164.26987) bodies 91 in component "Gas / Viewer-right exhaust fitting reference"
ref_plane "WorkPlane1" through (38.8, 0, 0) normal (1, 0, 0) x (0, 1, 0) in component "Chamber / AO2 face-seal allowance"
sketch "AO2 face seal allowance sketch" plane through (38.8, 0, 0) normal (1, 0, 0) x (0, 0, -1) in component "Chamber / AO2 face-seal allowance"
  circle A0 centre (-21.75, 142.5) radius 10.1
  dimension "d1919" = 21.75
  dimension "d1920" = 142.5
  dimension "d1921" = 10.1
  measures "d1919" horizontal distance of origin A0.centre
  measures "d1920" vertical distance of origin A0.centre
  measures "d1921" radius of A0
extrude "AO2 face seal allowance" add sketch "AO2 face seal allowance sketch" along normal blind 0.2 separate body contours A0 picked at (-24.531671, 144.396511) makes body 92 in component "Chamber / AO2 face-seal allowance"
ref_plane "WorkPlane2" through (38.7, 0, 0) normal (1, 0, 0) x (0, 1, 0) in component "Chamber / AO2 face-seal allowance"
sketch "AO2 face seal bore sketch" plane through (38.7, 0, 0) normal (1, 0, 0) x (0, 0, -1) in component "Chamber / AO2 face-seal allowance"
  circle A0 centre (-21.75, 142.5) radius 8
  dimension "d1926" = 21.75
  dimension "d1927" = 142.5
  dimension "d1928" = 8
  measures "d1926" horizontal distance of origin A0.centre
  measures "d1927" vertical distance of origin A0.centre
  measures "d1928" radius of A0
extrude "AO2 face seal bore" cut sketch "AO2 face seal bore sketch" along normal blind 0.4 contours A0 picked at (-25.326107, 141.166097) bodies 92 in component "Chamber / AO2 face-seal allowance"
ref_plane "WorkPlane1" through (0, 128.7, 0) normal (0, 1, 0) x (0, 0, 1) in component "Chamber / sealed harness feedthrough allowance"
sketch "Potted harness closure reference sketch" plane through (0, 128.7, 0) normal (0, 1, 0) x (1, 0, 0) in component "Chamber / sealed harness feedthrough allowance"
  circle A0 centre (17, -31.5) radius 2.2
  dimension "d1933" = 17
  dimension "d1934" = 31.5
  dimension "d1935" = 2.2
  measures "d1933" horizontal distance of origin A0.centre
  measures "d1934" vertical distance of origin A0.centre
  measures "d1935" radius of A0
extrude "Potted harness closure reference" add sketch "Potted harness closure reference sketch" along normal blind 3.3 separate body contours A0 picked at (17.227614, -32.642426) makes body 93 in component "Chamber / sealed harness feedthrough allowance"
ref_plane "WorkPlane29" through (0, 0, 22) normal (0, 0, 1) x (1, 0, 0) in component "Chamber / A3 top manifold with serial return"
sketch "Inlet elbow1 outerR4.5 semicircle" plane through (0, 0, 22) normal (0, 0, 1) x (1, 0, 0) in component "Chamber / A3 top manifold with serial return"
  arc A0 (70.75, 158) -> (70.75, 167) centre (70.75, 162.5) ccw
  line L0 (70.75, 158) -> (70.75, 167)
  point P0 (70.75, 162.5)
  dimension "d2164" = 70.75
  dimension "d2165" = 162.5
  dimension "d2166" = 4.5
  constraint vertical L0
  constraint vertical P0 A0.start
  constraint coincident P0 A0.centre
  measures "d2164" horizontal distance of origin A0.centre
  measures "d2165" vertical distance of origin A0.centre
  measures "d2166" radius of A0
revolve "Inlet elbow1 outerR4.5" add sketch "Inlet elbow1 outerR4.5 semicircle" angle 360 about axis through (70.75, 158, 22) along (0, 1, 0) contours A0 L0 picked at (72.911502, 162.661982) bodies 74 in component "Chamber / A3 top manifold with serial return"
ref_plane "WorkPlane30" through (0, 0, 22) normal (0, 0, 1) x (1, 0, 0) in component "Chamber / A3 top manifold with serial return"
sketch "Inlet elbow2 outerR4.5 semicircle" plane through (0, 0, 22) normal (0, 0, 1) x (1, 0, 0) in component "Chamber / A3 top manifold with serial return"
  arc A0 (70.75, 160.5) -> (70.75, 169.5) centre (70.75, 165) ccw
  line L0 (70.75, 160.5) -> (70.75, 169.5)
  point P0 (70.75, 165)
  dimension "d2170" = 70.75
  dimension "d2171" = 165
  dimension "d2172" = 4.5
  constraint vertical L0
  constraint vertical P0 A0.start
  constraint coincident P0 A0.centre
  measures "d2170" horizontal distance of origin A0.centre
  measures "d2171" vertical distance of origin A0.centre
  measures "d2172" radius of A0
revolve "Inlet elbow2 outerR4.5" add sketch "Inlet elbow2 outerR4.5 semicircle" angle 360 about axis through (70.75, 160.5, 22) along (0, 1, 0) contours A0 L0 picked at (71.842958, 163.581906) bodies 74 in component "Chamber / A3 top manifold with serial return"
ref_plane "WorkPlane31" through (0, 0, 22) normal (0, 0, 1) x (1, 0, 0) in component "Chamber / A3 top manifold with serial return"
sketch "Inlet elbow1 innerR2.5 semicircle" plane through (0, 0, 22) normal (0, 0, 1) x (1, 0, 0) in component "Chamber / A3 top manifold with serial return"
  arc A0 (70.75, 160) -> (70.75, 165) centre (70.75, 162.5) ccw
  line L0 (70.75, 160) -> (70.75, 165)
  point P0 (70.75, 162.5)
  dimension "d2176" = 70.75
  dimension "d2177" = 162.5
  dimension "d2178" = 2.5
  constraint vertical L0
  constraint vertical P0 A0.start
  constraint coincident P0 A0.centre
  measures "d2176" horizontal distance of origin A0.centre
  measures "d2177" vertical distance of origin A0.centre
  measures "d2178" radius of A0
revolve "Inlet elbow1 innerR2.5" cut sketch "Inlet elbow1 innerR2.5 semicircle" angle 360 about axis through (70.75, 160, 22) along (0, 1, 0) contours A0 L0 picked at (72.696061, 162.314566) bodies 74 in component "Chamber / A3 top manifold with serial return"
ref_plane "WorkPlane32" through (0, 0, 22) normal (0, 0, 1) x (1, 0, 0) in component "Chamber / A3 top manifold with serial return"
sketch "Inlet elbow2 innerR2.5 semicircle" plane through (0, 0, 22) normal (0, 0, 1) x (1, 0, 0) in component "Chamber / A3 top manifold with serial return"
  arc A0 (70.75, 162.5) -> (70.75, 167.5) centre (70.75, 165) ccw
  line L0 (70.75, 162.5) -> (70.75, 167.5)
  point P0 (70.75, 165)
  dimension "d2182" = 70.75
  dimension "d2183" = 165
  dimension "d2184" = 2.5
  constraint vertical L0
  constraint vertical P0 A0.start
  constraint coincident P0 A0.centre
  measures "d2182" horizontal distance of origin A0.centre
  measures "d2183" vertical distance of origin A0.centre
  measures "d2184" radius of A0
revolve "Inlet elbow2 innerR2.5" cut sketch "Inlet elbow2 innerR2.5 semicircle" angle 360 about axis through (70.75, 162.5, 22) along (0, 1, 0) contours A0 L0 picked at (72.696061, 164.814566) bodies 74 in component "Chamber / A3 top manifold with serial return"
ref_plane "WorkPlane33" through (0, 0, 22) normal (0, 0, 1) x (1, 0, 0) in component "Chamber / A3 top manifold with serial return"
sketch "Exhaust elbow1 innerR2.5 semicircle" plane through (0, 0, 22) normal (0, 0, 1) x (1, 0, 0) in component "Chamber / A3 top manifold with serial return"
  arc A0 (7.5, 160) -> (7.5, 165) centre (7.5, 162.5) ccw
  line L0 (7.5, 160) -> (7.5, 165)
  point P0 (7.5, 162.5)
  dimension "d2188" = 7.5
  dimension "d2189" = 162.5
  dimension "d2190" = 2.5
  constraint vertical L0
  constraint vertical P0 A0.start
  constraint coincident P0 A0.centre
  measures "d2188" horizontal distance of origin A0.centre
  measures "d2189" vertical distance of origin A0.centre
  measures "d2190" radius of A0
revolve "Exhaust elbow1 innerR2.5" cut sketch "Exhaust elbow1 innerR2.5 semicircle" angle 360 about axis through (7.5, 160, 22) along (0, 1, 0) contours A0 L0 picked at (8.191013, 161.879816) bodies 74 in component "Chamber / A3 top manifold with serial return"
ref_plane "WorkPlane34" through (0, 0, 33.5) normal (0, 0, 1) x (1, 0, 0) in component "Chamber / A3 top manifold with serial return"
sketch "Exhaust elbow2 innerR2.5 semicircle" plane through (0, 0, 33.5) normal (0, 0, 1) x (1, 0, 0) in component "Chamber / A3 top manifold with serial return"
  arc A0 (7.5, 160) -> (7.5, 165) centre (7.5, 162.5) ccw
  line L0 (7.5, 160) -> (7.5, 165)
  point P0 (7.5, 162.5)
  dimension "d2194" = 7.5
  dimension "d2195" = 162.5
  dimension "d2196" = 2.5
  constraint vertical L0
  constraint vertical P0 A0.start
  constraint coincident P0 A0.centre
  measures "d2194" horizontal distance of origin A0.centre
  measures "d2195" vertical distance of origin A0.centre
  measures "d2196" radius of A0
revolve "Exhaust elbow2 innerR2.5" cut sketch "Exhaust elbow2 innerR2.5 semicircle" angle 360 about axis through (7.5, 160, 33.5) along (0, 1, 0) contours A0 L0 picked at (8.191013, 161.879816) bodies 74 in component "Chamber / A3 top manifold with serial return"
combine "Join widened holder support to fixed divider" operation add target body 1 tool bodies 34 in component "01 Shape A housing"
ref_plane "WorkPlane35" through (70.65, 0, 0) normal (1, 0, 0) x (0, 1, 0) in component "Chamber / A3 top manifold with serial return"
sketch "Sketch35" plane through (70.65, 0, 0) normal (1, 0, 0) x (0, 0, -1) in component "Chamber / A3 top manifold with serial return"
  circle A0 centre (-22, 162.5) radius 2.5
  dimension "d2201" = 162.5
  dimension "d2202" = 2.5
  measures "d2201" vertical distance of origin A0.centre
  measures "d2202" radius of A0